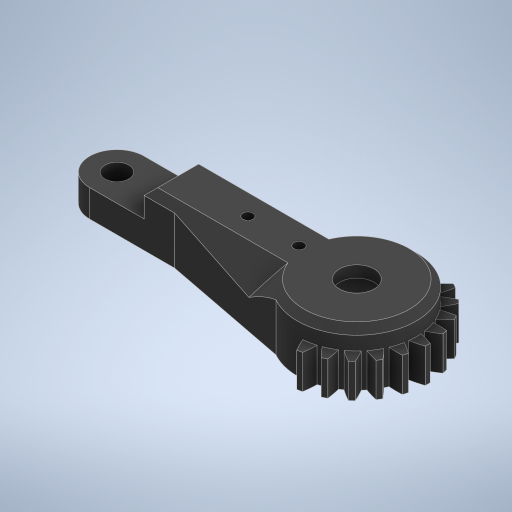
# Autodesk Inventor part: mechanism_1R
Saved by Autodesk Inventor 2023 (Build 270158000, 158)
## iProperties
Created: 2024-07-18
Part Number: mechanism_1R
Material: Generic
Document SubType Name: Modeling
Designer: Swoby
Density: 1 g/cm^3
Appearance: Default
Author: Swoby
Autodesk Inventor part; units mm, degrees
ref_plane "YZ Plane" through (0, 0, 0) normal (1, 0, 0) x (0, 1, 0)
ref_plane "XZ Plane" through (0, 0, 0) normal (0, 1, 0) x (-1, 0, 0)
ref_plane "XY Plane" through (0, 0, 0) normal (0, 0, 1) x (1, 0, 0)
sketch "Sketch1" plane through (0, 0, 0) normal (0, 1, 0) x (-1, 0, 0)
  circle A0 centre (0, 0) radius 1.75
  circle A1 centre (-35.232, 0) radius 6
  line L0 (0, 0) -> (-35.232, 0)
  line L1 (4, 0) -> (-39.232, 0) construction
  line L2 (0, -4) -> (-27.492, -4)
  line L3 (-35.232, 4) -> (-27.492, 4) construction
  arc A2 (0, -4) -> (0, 4) centre (0, 0) ccw
  arc A3 (-35.232, 4) -> (-35.232, -4) centre (-35.232, 0) ccw construction
  arc A4 (-26.5195, 0) -> (-27.492, 4) centre (-35.232, 0) ccw construction
  line L4 (-27.492, 4) -> (0, 4)
  arc A5 (-27.492, -4) -> (-26.5195, 0) centre (-35.232, 0) ccw construction
  arc A6 (-27.492, 4) -> (-27.492, -4) centre (-35.232, 0) ccw
  line L5 (-27.492, -4) -> (-35.232, -4) construction
  point P0 (-17.616, 0)
  dimension "d0" = 35.232
  dimension "d1" = 3.5
  dimension "d2" = 12
  dimension "d3" = 4
  dimension "d6" = 17.425
  constraints: 14 end point, 12 point on circle, 8 tangent, 7 centre point, 4 coincident, 4 parallel, 3 point on line, 2 horizontal, 1 midpoint
  measures "d0" distance of L0.end point (0, 0)
  measures "d1" diameter of A0
  measures "d2" diameter of A1
  measures "d3" radius of A2
  measures "d6" diameter of A4
extrude "Extrusion1" add sketch "Sketch1" along normal blind 4 contours A1 | L2 A6 L4 A2
sketch "Sketch2" plane through (0, 4, 0) normal (0, 1, 0) x (1, 0, 0)
  circle A0 centre (35.232, 0) radius 8.7125
  arc A1 (27.492, -4) -> (27.492, 4) centre (35.232, 0) ccw projected
  point P0 (0, 0)
  constraints: 1 coincident, 3 other
extrude "Extrusion2" add sketch "Sketch2" along normal blind 4
sketch "Sketch3" plane through (0, 0, 0) normal (0, -1, 0) x (1, 0, 0)
  line L0 (35.232, 0) -> (0, 0) construction
  line L1 (35.232, 0) -> (35.232, 10.5885) construction
  line L2 (35.232, 0) -> (40.5262, -9.1699) construction
  arc A0 (27.492, -4) -> (27.492, 4) centre (35.232, 0) ccw projected
  arc A1 (40.5262, -9.1699) -> (39.9268, -9.4908) centre (35.232, 0) ccw construction
  arc A2 (40.6031, -6.8599) -> (40.1229, -7.2102) centre (35.232, 0) ccw construction
  line L3 (35.232, 0) -> (43.9115, -0.7578) construction
  line L4 (35.232, 0) -> (43.8396, -1.3479) construction
  line L5 (35.232, 0) -> (43.8841, 1.024) construction
  line L6 (35.232, 0) -> (45.8075, 0.5246) construction
  line L7 (35.232, 0) -> (45.8186, -0.1996) construction
  arc A3 (45.8075, 0.5246) -> (43.8841, 1.024) centre (41.1455, -13.4766) ccw
  arc A4 (43.9115, -0.7578) -> (45.8186, -0.1996) centre (40.7288, 13.6519) ccw
  arc A5 (45.8186, -0.1996) -> (45.8075, 0.5246) centre (35.232, 0) ccw
  arc A6 (43.8396, -1.3479) -> (43.9115, -0.7578) centre (35.232, 0) ccw
  line L8 (35.232, 0) -> (43.2871, 3.3201) construction
  line L9 (35.232, 0) -> (43.7941, 1.6116) construction
  line L10 (35.232, 0) -> (45.2739, 3.358) construction
  line L11 (35.232, 0) -> (45.48, 2.6637) construction
  arc A7 (43.7941, 1.6116) -> (43.2871, 3.3201) centre (35.232, 0) ccw construction
  arc A8 (43.8841, 1.024) -> (43.7941, 1.6116) centre (35.232, 0) ccw
  arc A9 (45.48, 2.6637) -> (45.2739, 3.358) centre (35.232, 0) ccw
  arc A10 (45.2739, 3.358) -> (44.3815, 5.3294) centre (35.232, 0) ccw construction
  arc A11 (43.7941, 1.6116) -> (45.48, 2.6637) centre (36.8423, 14.6286) ccw
  arc A12 (45.2739, 3.358) -> (43.2871, 3.3201) centre (44.5617, -11.3818) ccw
  line L12 (35.232, 0) -> (43.042, 3.8616) construction
  line L13 (35.232, 0) -> (44.3815, 5.3294) construction
  line L14 (35.232, 0) -> (43.9958, 5.9424) construction
  line L15 (35.232, 0) -> (42.0929, 5.3699) construction
  arc A13 (44.3815, 5.3294) -> (43.9958, 5.9424) centre (35.232, 0) ccw
  arc A14 (43.9958, 5.9424) -> (42.6047, 7.6) centre (35.232, 0) ccw construction
  arc A15 (43.042, 3.8616) -> (42.0929, 5.3699) centre (35.232, 0) ccw construction
  arc A16 (43.2871, 3.3201) -> (43.042, 3.8616) centre (35.232, 0) ccw
  arc A17 (42.0929, 5.3699) -> (41.7107, 5.8253) centre (35.232, 0) ccw
  arc A18 (43.042, 3.8616) -> (44.3815, 5.3294) centre (32.8364, 14.5206) ccw
  arc A19 (43.9958, 5.9424) -> (42.0929, 5.3699) centre (47.2862, -8.443) ccw
  line L16 (35.232, 0) -> (41.7107, 5.8253) construction
  line L17 (35.232, 0) -> (42.6047, 7.6) construction
  line L18 (35.232, 0) -> (42.0678, 8.0863) construction
  line L19 (35.232, 0) -> (40.3899, 7.0217) construction
  line L20 (35.232, 0) -> (39.8991, 7.357) construction
  line L21 (35.232, 0) -> (40.2811, 9.3071) construction
  line L22 (35.232, 0) -> (39.6331, 9.6305) construction
  line L23 (35.232, 0) -> (38.3045, 8.1527) construction
  arc A20 (41.7107, 5.8253) -> (40.3899, 7.0217) centre (35.232, 0) ccw construction
  arc A21 (39.8991, 7.357) -> (38.3045, 8.1527) centre (35.232, 0) ccw construction
  arc A22 (40.3899, 7.0217) -> (39.8991, 7.357) centre (35.232, 0) ccw
  arc A23 (38.3045, 8.1527) -> (37.7415, 8.3433) centre (35.232, 0) ccw
  arc A24 (40.2811, 9.3071) -> (39.6331, 9.6305) centre (35.232, 0) ccw
  arc A25 (39.6331, 9.6305) -> (37.5833, 10.3241) centre (35.232, 0) ccw construction
  arc A26 (42.0678, 8.0863) -> (40.2811, 9.3071) centre (35.232, 0) ccw construction
  arc A27 (42.6047, 7.6) -> (42.0678, 8.0863) centre (35.232, 0) ccw
  arc A28 (39.6331, 9.6305) -> (38.3045, 8.1527) centre (49.9181, -0.9519) ccw
  arc A29 (39.8991, 7.357) -> (40.2811, 9.3071) centre (25.6413, 11.1627) ccw
  arc A30 (42.0678, 8.0863) -> (40.3899, 7.0217) centre (49.1169, -4.8783) ccw
  arc A31 (41.7107, 5.8253) -> (42.6047, 7.6) centre (29.0081, 13.3361) ccw
  line L24 (35.232, 0) -> (37.7415, 8.3433) construction
  line L25 (35.232, 0) -> (37.5833, 10.3241) construction
  line L26 (35.232, 0) -> (36.872, 10.4607) construction
  line L27 (35.232, 0) -> (35.9913, 8.6793) construction
  arc A32 (37.7415, 8.3433) -> (35.232, 8.7125) centre (35.232, 0) ccw construction
  arc A33 (37.5833, 10.3241) -> (36.872, 10.4607) centre (35.232, 0) ccw
  arc A34 (36.872, 10.4607) -> (35.232, 10.5885) centre (35.232, 0) ccw construction
  arc A35 (36.872, 10.4607) -> (35.9913, 8.6793) centre (49.6304, 3.0452) ccw
  arc A36 (37.7415, 8.3433) -> (37.5833, 10.3241) centre (22.9856, 8.1617) ccw
  line L28 (35.232, 0) -> (45.557, -2.3477) construction
  line L29 (35.232, 0) -> (45.3723, -3.048) construction
  line L30 (35.232, 0) -> (43.3853, -3.0711) construction
  line L31 (35.232, 0) -> (43.1569, -3.6199) construction
  line L32 (35.232, 0) -> (44.5409, -5.0459) construction
  line L33 (35.232, 0) -> (44.1741, -5.6705) construction
  line L34 (35.232, 0) -> (42.2546, -5.1567) construction
  line L35 (35.232, 0) -> (41.8866, -5.6236) construction
  line L36 (35.232, 0) -> (42.8346, -7.37) construction
  line L37 (35.232, 0) -> (42.313, -7.8725) construction
  line L38 (35.232, 0) -> (40.6031, -6.8599) construction
  line L39 (35.232, 0) -> (40.1229, -7.2102) construction
  line L40 (35.232, 0) -> (40.5646, -9.1477) construction
  line L41 (35.232, 0) -> (39.9268, -9.4908) construction
  line L42 (35.232, 0) -> (38.5535, -8.0545) construction
  arc A37 (45.557, -2.3477) -> (43.8396, -1.3479) centre (37.2908, -14.5722) ccw
  arc A38 (45.557, -2.3477) -> (45.48, 2.6637) centre (35.232, 0) ccw construction
  arc A39 (45.3723, -3.048) -> (45.557, -2.3477) centre (35.232, 0) ccw
  arc A40 (43.3853, -3.0711) -> (43.8841, 1.024) centre (35.232, 0) ccw construction
  arc A41 (43.1569, -3.6199) -> (43.3853, -3.0711) centre (35.232, 0) ccw
  arc A42 (44.1741, -5.6705) -> (44.5409, -5.0459) centre (35.232, 0) ccw
  arc A43 (44.5409, -5.0459) -> (45.3723, -3.048) centre (35.232, 0) ccw construction
  arc A44 (42.313, -7.8725) -> (42.8346, -7.37) centre (35.232, 0) ccw
  arc A45 (42.8346, -7.37) -> (44.1741, -5.6705) centre (35.232, 0) ccw construction
  arc A46 (39.9268, -9.4908) -> (40.5646, -9.1477) centre (35.232, 0) ccw
  arc A47 (40.5646, -9.1477) -> (42.313, -7.8725) centre (35.232, 0) ccw construction
  arc A48 (41.8866, -5.6236) -> (42.2546, -5.1567) centre (35.232, 0) ccw
  arc A49 (42.2546, -5.1567) -> (43.1569, -3.6199) centre (35.232, 0) ccw construction
  arc A50 (40.6031, -6.8599) -> (41.8866, -5.6236) centre (35.232, 0) ccw construction
  arc A51 (40.1229, -7.2102) -> (40.6031, -6.8599) centre (35.232, 0) ccw
  arc A52 (43.3853, -3.0711) -> (45.3723, -3.048) centre (44.2077, 11.6629) ccw
  arc A53 (44.5409, -5.0459) -> (43.1569, -3.6199) centre (33.2835, -14.5874) ccw
  arc A54 (42.2546, -5.1567) -> (44.1741, -5.6705) centre (47.0212, 8.8093) ccw
  arc A55 (42.8346, -7.37) -> (41.8866, -5.6236) centre (29.4206, -13.5209) ccw
  arc A56 (40.6031, -6.8599) -> (42.313, -7.8725) centre (48.9605, 5.3024) ccw
  arc A57 (40.5646, -9.1477) -> (40.1229, -7.2102) centre (25.9886, -11.452) ccw
  arc A58 (38.5535, -8.0545) -> (39.9268, -9.4908) centre (49.882, 1.4025) ccw
  line L43 (35.232, 0) -> (35.9913, 8.6793)
  point P0 (40.1229, -7.2102)
  point P1 (41.8866, -5.6236)
  point P2 (43.1569, -3.6199)
  point P3 (42.2546, -5.1567)
  point P4 (43.8396, -1.3479)
  point P5 (43.3853, -3.0711)
  point P6 (43.8841, 1.024)
  point P7 (43.9115, -0.7578)
  point P8 (43.2871, 3.3201)
  point P9 (43.7941, 1.6116)
  point P10 (42.0929, 5.3699)
  point P11 (43.042, 3.8616)
  point P12 (40.3899, 7.0217)
  point P13 (41.7107, 5.8253)
  point P14 (38.3045, 8.1527)
  point P15 (39.8991, 7.357)
  point P16 (35.9913, 8.6793)
  dimension "d12" = 90
  dimension "d13" = 150
  dimension "d23" = 10.5885
  dimension "d26" = 11.74
  dimension "d27" = 3.91
  dimension "d28" = 3.91
  dimension "d29" = 14.757
  dimension "d30" = 14.757
  dimension "d31" = 10.5885
  dimension "d33" = 3.91
  dimension "d34" = 3.91
  dimension "d35" = 3.91
  dimension "d36" = 11.74
  dimension "d37" = 14.757
  dimension "d38" = 14.757
  dimension "d39" = 3.91
  dimension "d40" = 3.91
  dimension "d41" = 3.91
  dimension "d42" = 11.74
  dimension "d43" = 14.757
  dimension "d44" = 14.757
  dimension "d45" = 3.91
  dimension "d46" = 3.91
  dimension "d47" = 3.91
  dimension "d48" = 11.74
  dimension "d49" = 3.91
  dimension "d50" = 3.91
  dimension "d51" = 11.74
  dimension "d52" = 3.91
  dimension "d54" = 14.757
  dimension "d55" = 14.757
  dimension "d56" = 14.757
  dimension "d57" = 14.757
  dimension "d58" = 3.91
  dimension "d59" = 3.91
  dimension "d60" = 11.74
  dimension "d61" = 3.91
  dimension "d62" = 14.757
  dimension "d63" = 14.757
  dimension "d64" = 3.91
  dimension "d65" = 3.91
  dimension "d66" = 11.74
  dimension "d67" = 3.91
  dimension "d68" = 3.91
  dimension "d69" = 3.91
  dimension "d70" = 11.74
  dimension "d71" = 3.91
  dimension "d72" = 3.91
  dimension "d74" = 3.91
  dimension "d75" = 11.74
  dimension "d76" = 3.91
  dimension "d77" = 3.91
  dimension "d78" = 3.91
  dimension "d79" = 11.74
  dimension "d81" = 14.757
  dimension "d82" = 14.757
  dimension "d83" = 14.757
  dimension "d84" = 14.757
  dimension "d85" = 14.757
  dimension "d86" = 14.757
  dimension "d87" = 14.757
  dimension "d88" = 14.757
  dimension "d91" = 3.91
  dimension "d92" = 95
  constraints: 172 point on circle, 57 centre point, 43 end point, 1 concentric, 1 vertical alignment, 62 other
  measures "d23" radius of A1
  measures "d26" angle of L3 L5
  measures "d27" angle of L6 L5
  measures "d28" angle of L3 L7
  measures "d29" radius of A3
  measures "d30" radius of A4
  measures "d31" radius of A5
  measures "d33" angle of L5 L9
  measures "d34" angle of L9 L11
  measures "d35" angle of L10 L8
  measures "d36" angle of L9 L8
  measures "d37" radius of A12
  measures "d38" radius of A11
  measures "d39" angle of L8 L12
  measures "d40" angle of L12 L13
  measures "d41" angle of L14 L15
  measures "d42" angle of L12 L15
  measures "d43" radius of A19
  measures "d44" radius of A18
  measures "d45" angle of L15 L16
  measures "d46" angle of L18 L19
  measures "d47" angle of L16 L17
  measures "d48" angle of L16 L19
  measures "d49" angle of L21 L20
  measures "d50" angle of L23 L22
  measures "d51" angle of L20 L23
  measures "d52" angle of L19 L20
  measures "d54" radius of A30
  measures "d55" radius of A31
  measures "d56" radius of A29
  measures "d57" radius of A28
  measures "d58" angle of L23 L24
  measures "d59" angle of L25 L24
  measures "d60" angle of L27 L24
  measures "d61" angle of L26 L27
  measures "d62" radius of A36
  measures "d63" radius of A35
  measures "d64" angle of L28 L4
  measures "d65" angle of L30 L29
  measures "d66" angle of L4 L30
  measures "d67" angle of L31 L30
  measures "d68" angle of L31 L32
  measures "d69" angle of L33 L34
  measures "d70" angle of L31 L34
  measures "d71" angle of L34 L35
  measures "d72" angle of L35 L36
  measures "d74" angle of L37 L38
  measures "d75" angle of L35 L38
  measures "d76" angle of L39 L38
  measures "d77" angle of L39 L40
  measures "d78" angle of L41 L42
  measures "d79" angle of L39 L42
  measures "d81" radius of A37
  measures "d82" radius of A52
  measures "d83" radius of A53
  measures "d84" radius of A54
  measures "d85" radius of A55
  measures "d86" radius of A56
  measures "d87" radius of A57
  measures "d88" radius of A58
  measures "d91" angle of L4 L3
  measures "d92" angle to the sketch x axis of L43
extrude "Extrusion3" add sketch "Sketch3" against normal blind 5
sketch "Sketch4" plane through (0, 0, 0) normal (0, -1, 0) x (1, 0, 0)
  arc A0 (35.9913, 8.6793) -> (27.492, 4) centre (35.232, 0) ccw projected
  arc A1 (34.9224, -3.5867) -> (34.9224, 3.5867) centre (35.232, 0) ccw
  arc A2 (19.3385, 2.2417) -> (19.3385, -2.2417) centre (19.532, 0) ccw
  line L0 (19.532, 0) -> (38.832, 0) construction
  line L1 (19.3385, 2.2417) -> (34.9224, 3.5867)
  line L2 (19.3385, -2.2417) -> (34.9224, -3.5867)
  line L3 (17.282, 0) -> (19.532, 0) construction
  arc A3 (21.782, 0) -> (19.3385, 2.2417) centre (19.532, 0) ccw construction
  arc A4 (19.3385, -2.2417) -> (21.782, 0) centre (19.532, 0) ccw construction
  arc A5 (31.632, 0) -> (34.9224, -3.5867) centre (35.232, 0) ccw construction
  arc A6 (34.9224, 3.5867) -> (31.632, 0) centre (35.232, 0) ccw construction
  line L4 (34.8623, 4.2841) -> (19.2783, 2.9391)
  arc A7 (19.2783, 2.9391) -> (19.2783, -2.9391) centre (19.532, 0) ccw
  line L5 (19.2783, -2.9391) -> (34.8623, -4.2841)
  arc A8 (34.8623, -4.2841) -> (34.8623, 4.2841) centre (35.232, 0) ccw
  point P0 (0, 0)
  dimension "d93" = 7.2
  dimension "d94" = 4.5
  dimension "d97" = 15.7
  dimension "d98" = 0.7
  constraints: 20 point on circle, 12 end point, 8 centre point, 8 tangent, 3 point on line, 2 horizontal, 1 coincident, 3 other
  measures "d93" diameter of A1
  measures "d94" diameter of A2
  measures "d97" distance of A0.centre L0.start
  measures "d98" distance between parallel lines of L1 L4
sketch "Sketch5" plane through (0, 4, 0) normal (0, 1, 0) x (1, 0, 0)
  circle A0 centre (0, 0) radius 1.75 projected
  arc A1 (27.492, 4) -> (27.492, -4) centre (35.232, 0) ccw projected
  line L0 (27.492, 4) -> (0, 4) projected
  arc A2 (0, 4) -> (0, -4) centre (0, 0) ccw projected
  line L1 (0, -4) -> (27.492, -4) projected
  line L2 (8, 4) -> (8, -4)
  dimension "d99" = 8
  constraints: 2 end point, 2 point on line, 1 perpendicular
  measures "d99" distance from line of L2 point (0, 0)
extrude "Extrusion4" add sketch "Sketch5" along normal up to surface (4 mm away) contours A1 L1 L2 L0
chamfer "Chamfer2" distance 1 angle 45 5 edges at (37.2903, 8, 8.4659) (37.2903, 8, -8.4659) (17.746, 8, 4) (17.746, 8, -4) (8, 8, 0)
extrude "Extrusion5" cut sketch "Sketch4" against normal blind 6.3 contours L2 A2 L1 A1 | A8 L5 A7 L4
sketch "Sketch6" plane through (0, 6.3, 0) normal (0, -1, 0) x (1, 0, 0)
  arc A0 (34.8623, -4.2841) -> (34.8623, 4.2841) centre (35.232, 0) ccw projected
  circle A1 centre (35.232, 0) radius 2.55
  point P0 (0, 0)
  dimension "d107" = 5.1
  constraints: 1 centre point, 1 coincident
  measures "d107" diameter of A1
extrude "Extrusion6" cut sketch "Sketch6" against normal through all
chamfer "Chamfer3" distance 15 distance2 5 2 edges at (27.492, 5.5, 4) (27.492, 2, 4) measured on face at (26.992, 2, 4) measured on face at (26.992, 5.5, 4)
chamfer "Chamfer4" distance 5 distance2 15 1 edges at (27.492, 3.5, -4) measured on face at (27.7339, 3.5, -4.4369)
sketch "Sketch7" plane through (0, 6.3, 0) normal (0, -1, 0) x (1, 0, 0)
  circle A0 centre (35.232, 0) radius 2.55 projected
  circle A1 centre (35.232, 0) radius 4.3
  arc A2 (34.8623, -4.2841) -> (34.8623, 4.2841) centre (35.232, 0) ccw projected
  circle A3 centre (35.232, 0) radius 6.3
  circle A4 centre (35.232, 0) radius 2.55 projected
  arc A5 (19.2783, 2.9391) -> (19.2783, -2.9391) centre (19.532, 0) ccw projected
  line L0 (34.8623, -4.2841) -> (19.2783, -2.9391) projected
  arc A6 (34.8623, -4.2841) -> (34.8623, 4.2841) centre (35.232, 0) ccw projected
  line L1 (19.2783, 2.9391) -> (34.8623, 4.2841) projected
  point P0 (0, 0)
  point P1 (30.275, -3.8882)
  point P2 (30.275, 3.8882)
  dimension "d116" = 2
  constraints: 1 centre point, 1 coincident, 3 other
extrude "Extrusion7" add sketch "Sketch7" along normal blind 1.4 contours A3 L0 A5 L1
chamfer "Chamfer5" distance 1.4 angle 45 1 edges at (28.932, 4.9, 0)
sketch "Sketch8" plane through (0, 4.9, 0) normal (0, -1, 0) x (1, 0, 0)
  circle A0 centre (19.232, 0) radius 0.75
  circle A1 centre (35.232, 0) radius 2.55 projected
  circle A2 centre (26.732, 0) radius 0.75
  line L0 (19.232, 0) -> (35.232, 0)
  point P0 (0, 0)
  dimension "d122" = 1.5
  dimension "d123" = 16
  dimension "d126" = 1.5
  dimension "d127" = 8.5
  constraints: 2 centre point, 2 end point, 1 horizontal, 1 point on line
  measures "d122" diameter of A0
  measures "d123" distance of L0.end L0.start
  measures "d126" diameter of A2
  measures "d127" distance of L0.end A2.centre
extrude "Extrusion8" cut sketch "Sketch8" against normal blind 4 contours A0 | L0 A2 | A2 L0
equation "\"d31\" = d23"
equation "\"d37\" = d29"
equation "\"d38\" = d30"
equation "\"d42\" = d36"
equation "\"d43\" = d30"
equation "\"d44\" = d38"
equation "\"d45\" = d41"
equation "\"d46\" = d45"
equation "\"d47\" = d45"
equation "\"d48\" = d36"
equation "\"d49\" = d47"
equation "\"d50\" = d49"
equation "\"d51\" = d48"
equation "\"d54\" = d43"
equation "\"d55\" = d54"
equation "\"d56\" = d55"
equation "\"d57\" = d55"
equation "\"d62\" = d56"
equation "\"d63\" = d56"
body "Solid1"
